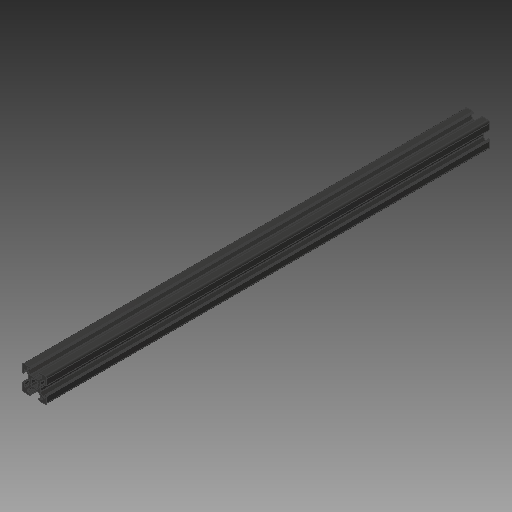
# Autodesk Inventor part: Profile horizontal 20x20x360
Saved by Autodesk Inventor 2017 (Build 210142000, 142)
## iProperties
Company: FABLAB Frenchmakers
Part Number: Profile horizontal 20x20x360
Material: Aluminium
Document SubType Name: Modeling
Designer: FABLAB Frenchmakers
Density: 2.7 g/cm^3
Appearance: Aluminium - Plat(1)
Mass: 157.502 g
Surface Area: 633.6 cm^2
Volume: 58.3342 cm^3
Stock Number: 1420-01-03
Project: 1420 Vauban 3D XL
Catalog Web Link: http://frenchmakers.com/
Autodesk Inventor part; units mm, degrees
ref_plane "YZ Plane" through (0, 0, 0) normal (1, 0, 0) x (0, 1, 0)
ref_plane "XZ Plane" through (0, 0, 0) normal (0, 1, 0) x (-1, 0, 0)
ref_plane "XY Plane" through (0, 0, 0) normal (0, 0, 1) x (1, 0, 0)
sketch "Esquisse1" plane through (0, 0, 0) normal (0, 0, 1) x (1, 0, 0)
  arc A0 (10, 8.5) -> (8.5, 10) centre (8.5, 8.5) ccw
  line L0 (3.85, 10) -> (8.5, 10)
  arc A1 (3.85, 10) -> (3.65, 9.8) centre (3.85, 9.8) ccw
  line L1 (3.65, 9.5) -> (3.65, 9.8)
  line L2 (3.3, 9.5) -> (3.65, 9.5)
  arc A2 (3.3, 9.5) -> (3.1, 9.3) centre (3.3, 9.3) ccw
  line L3 (3.1, 9) -> (3.1, 9.3)
  arc A3 (3.1, 9) -> (3.6, 8.5) centre (3.6, 9) ccw
  line L4 (5.5, 8.5) -> (3.6, 8.5)
  arc A4 (6, 8) -> (5.5, 8.5) centre (5.5, 8) ccw
  line L5 (6, 7.2678) -> (6, 8)
  arc A5 (5.8536, 6.9142) -> (6, 7.2678) centre (5.5, 7.2678) ccw
  line L6 (3.5858, 4.6464) -> (5.8536, 6.9142)
  arc A6 (3.2322, 4.5) -> (3.5858, 4.6464) centre (3.2322, 5) ccw
  line L7 (0.9536, 4.5) -> (3.2322, 4.5)
  arc A7 (0.9536, 4.5) -> (0.8536, 4.4732) centre (0.9536, 4.3) ccw
  line L8 (0.1, 4.0381) -> (0.8536, 4.4732)
  arc A8 (-0.1, 4.0381) -> (0.1, 4.0381) centre (0, 4.2113) ccw
  line L9 (-0.8536, 4.4732) -> (-0.1, 4.0381)
  arc A9 (-0.8536, 4.4732) -> (-0.9536, 4.5) centre (-0.9536, 4.3) ccw
  line L10 (-3.2322, 4.5) -> (-0.9536, 4.5)
  arc A10 (-3.5858, 4.6464) -> (-3.2322, 4.5) centre (-3.2322, 5) ccw
  line L11 (-5.8536, 6.9142) -> (-3.5858, 4.6464)
  arc A11 (-6, 7.2678) -> (-5.8536, 6.9142) centre (-5.5, 7.2678) ccw
  line L12 (-6, 8) -> (-6, 7.2678)
  arc A12 (-5.5, 8.5) -> (-6, 8) centre (-5.5, 8) ccw
  line L13 (-3.6, 8.5) -> (-5.5, 8.5)
  arc A13 (-3.6, 8.5) -> (-3.1, 9) centre (-3.6, 9) ccw
  line L14 (-3.1, 9.3) -> (-3.1, 9)
  arc A14 (-3.1, 9.3) -> (-3.3, 9.5) centre (-3.3, 9.3) ccw
  line L15 (-3.65, 9.5) -> (-3.3, 9.5)
  line L16 (-3.65, 9.8) -> (-3.65, 9.5)
  arc A15 (-3.65, 9.8) -> (-3.85, 10) centre (-3.85, 9.8) ccw
  line L17 (-8.5, 10) -> (-3.85, 10)
  arc A16 (-8.5, 10) -> (-10, 8.5) centre (-8.5, 8.5) ccw
  line L18 (-10, 3.85) -> (-10, 8.5)
  arc A17 (-10, 3.85) -> (-9.8, 3.65) centre (-9.8, 3.85) ccw
  line L19 (-9.5, 3.65) -> (-9.8, 3.65)
  line L20 (-9.5, 3.3) -> (-9.5, 3.65)
  arc A18 (-9.5, 3.3) -> (-9.3, 3.1) centre (-9.3, 3.3) ccw
  line L21 (-9, 3.1) -> (-9.3, 3.1)
  arc A19 (-9, 3.1) -> (-8.5, 3.6) centre (-9, 3.6) ccw
  line L22 (-8.5, 5.5) -> (-8.5, 3.6)
  arc A20 (-8, 6) -> (-8.5, 5.5) centre (-8, 5.5) ccw
  line L23 (-7.2678, 6) -> (-8, 6)
  arc A21 (-6.9142, 5.8536) -> (-7.2678, 6) centre (-7.2678, 5.5) ccw
  line L24 (-4.6464, 3.5858) -> (-6.9142, 5.8536)
  arc A22 (-4.5, 3.2322) -> (-4.6464, 3.5858) centre (-5, 3.2322) ccw
  line L25 (-4.5, 0.9536) -> (-4.5, 3.2322)
  arc A23 (-4.5, 0.9536) -> (-4.4732, 0.8536) centre (-4.3, 0.9536) ccw
  line L26 (-4.0381, 0.1) -> (-4.4732, 0.8536)
  arc A24 (-4.0381, -0.1) -> (-4.0381, 0.1) centre (-4.2113, 0) ccw
  line L27 (-4.4732, -0.8536) -> (-4.0381, -0.1)
  arc A25 (-4.4732, -0.8536) -> (-4.5, -0.9536) centre (-4.3, -0.9536) ccw
  line L28 (-4.5, -3.2322) -> (-4.5, -0.9536)
  arc A26 (-4.6464, -3.5858) -> (-4.5, -3.2322) centre (-5, -3.2322) ccw
  line L29 (-6.9142, -5.8536) -> (-4.6464, -3.5858)
  arc A27 (-7.2678, -6) -> (-6.9142, -5.8536) centre (-7.2678, -5.5) ccw
  line L30 (-8, -6) -> (-7.2678, -6)
  arc A28 (-8.5, -5.5) -> (-8, -6) centre (-8, -5.5) ccw
  line L31 (-8.5, -3.6) -> (-8.5, -5.5)
  arc A29 (-8.5, -3.6) -> (-9, -3.1) centre (-9, -3.6) ccw
  line L32 (-9.3, -3.1) -> (-9, -3.1)
  arc A30 (-9.3, -3.1) -> (-9.5, -3.3) centre (-9.3, -3.3) ccw
  line L33 (-9.5, -3.65) -> (-9.5, -3.3)
  line L34 (-9.8, -3.65) -> (-9.5, -3.65)
  arc A31 (-9.8, -3.65) -> (-10, -3.85) centre (-9.8, -3.85) ccw
  line L35 (-10, -8.5) -> (-10, -3.85)
  arc A32 (-10, -8.5) -> (-8.5, -10) centre (-8.5, -8.5) ccw
  line L36 (-3.85, -10) -> (-8.5, -10)
  arc A33 (-3.85, -10) -> (-3.65, -9.8) centre (-3.85, -9.8) ccw
  line L37 (-3.65, -9.5) -> (-3.65, -9.8)
  line L38 (-3.3, -9.5) -> (-3.65, -9.5)
  arc A34 (-3.3, -9.5) -> (-3.1, -9.3) centre (-3.3, -9.3) ccw
  line L39 (-3.1, -9) -> (-3.1, -9.3)
  arc A35 (-3.1, -9) -> (-3.6, -8.5) centre (-3.6, -9) ccw
  line L40 (-5.5, -8.5) -> (-3.6, -8.5)
  arc A36 (-6, -8) -> (-5.5, -8.5) centre (-5.5, -8) ccw
  line L41 (-6, -7.2678) -> (-6, -8)
  arc A37 (-5.8536, -6.9142) -> (-6, -7.2678) centre (-5.5, -7.2678) ccw
  line L42 (-3.5858, -4.6464) -> (-5.8536, -6.9142)
  arc A38 (-3.2322, -4.5) -> (-3.5858, -4.6464) centre (-3.2322, -5) ccw
  line L43 (-0.9536, -4.5) -> (-3.2322, -4.5)
  arc A39 (-0.9536, -4.5) -> (-0.8536, -4.4732) centre (-0.9536, -4.3) ccw
  line L44 (-0.1, -4.0381) -> (-0.8536, -4.4732)
  arc A40 (0.1, -4.0381) -> (-0.1, -4.0381) centre (0, -4.2113) ccw
  line L45 (0.8536, -4.4732) -> (0.1, -4.0381)
  arc A41 (0.8536, -4.4732) -> (0.9536, -4.5) centre (0.9536, -4.3) ccw
  line L46 (3.2322, -4.5) -> (0.9536, -4.5)
  arc A42 (3.5858, -4.6464) -> (3.2322, -4.5) centre (3.2322, -5) ccw
  line L47 (5.8536, -6.9142) -> (3.5858, -4.6464)
  arc A43 (6, -7.2678) -> (5.8536, -6.9142) centre (5.5, -7.2678) ccw
  line L48 (6, -8) -> (6, -7.2678)
  arc A44 (5.5, -8.5) -> (6, -8) centre (5.5, -8) ccw
  line L49 (3.6, -8.5) -> (5.5, -8.5)
  arc A45 (3.6, -8.5) -> (3.1, -9) centre (3.6, -9) ccw
  line L50 (3.1, -9.3) -> (3.1, -9)
  arc A46 (3.1, -9.3) -> (3.3, -9.5) centre (3.3, -9.3) ccw
  line L51 (3.65, -9.5) -> (3.3, -9.5)
  line L52 (3.65, -9.8) -> (3.65, -9.5)
  arc A47 (3.65, -9.8) -> (3.85, -10) centre (3.85, -9.8) ccw
  line L53 (8.5, -10) -> (3.85, -10)
  arc A48 (8.5, -10) -> (10, -8.5) centre (8.5, -8.5) ccw
  line L54 (10, -3.85) -> (10, -8.5)
  arc A49 (10, -3.85) -> (9.8, -3.65) centre (9.8, -3.85) ccw
  line L55 (9.5, -3.65) -> (9.8, -3.65)
  line L56 (9.5, -3.3) -> (9.5, -3.65)
  arc A50 (9.5, -3.3) -> (9.3, -3.1) centre (9.3, -3.3) ccw
  line L57 (9, -3.1) -> (9.3, -3.1)
  arc A51 (9, -3.1) -> (8.5, -3.6) centre (9, -3.6) ccw
  line L58 (8.5, -5.5) -> (8.5, -3.6)
  arc A52 (8, -6) -> (8.5, -5.5) centre (8, -5.5) ccw
  line L59 (7.2678, -6) -> (8, -6)
  arc A53 (6.9142, -5.8536) -> (7.2678, -6) centre (7.2678, -5.5) ccw
  line L60 (4.6464, -3.5858) -> (6.9142, -5.8536)
  arc A54 (4.5, -3.2322) -> (4.6464, -3.5858) centre (5, -3.2322) ccw
  line L61 (4.5, -0.9536) -> (4.5, -3.2322)
  arc A55 (4.5, -0.9536) -> (4.4732, -0.8536) centre (4.3, -0.9536) ccw
  line L62 (4.0381, -0.1) -> (4.4732, -0.8536)
  arc A56 (4.0381, 0.1) -> (4.0381, -0.1) centre (4.2113, 0) ccw
  line L63 (4.4732, 0.8536) -> (4.0381, 0.1)
  arc A57 (4.4732, 0.8536) -> (4.5, 0.9536) centre (4.3, 0.9536) ccw
  line L64 (4.5, 3.2322) -> (4.5, 0.9536)
  arc A58 (4.6464, 3.5858) -> (4.5, 3.2322) centre (5, 3.2322) ccw
  line L65 (6.9142, 5.8536) -> (4.6464, 3.5858)
  arc A59 (7.2678, 6) -> (6.9142, 5.8536) centre (7.2678, 5.5) ccw
  line L66 (8, 6) -> (7.2678, 6)
  arc A60 (8.5, 5.5) -> (8, 6) centre (8, 5.5) ccw
  line L67 (8.5, 3.6) -> (8.5, 5.5)
  arc A61 (8.5, 3.6) -> (9, 3.1) centre (9, 3.6) ccw
  line L68 (9.3, 3.1) -> (9, 3.1)
  arc A62 (9.3, 3.1) -> (9.5, 3.3) centre (9.3, 3.3) ccw
  line L69 (9.5, 3.65) -> (9.5, 3.3)
  line L70 (9.8, 3.65) -> (9.5, 3.65)
  arc A63 (9.8, 3.65) -> (10, 3.85) centre (9.8, 3.85) ccw
  line L71 (10, 8.5) -> (10, 3.85)
  arc A64 (2.9922, 1.9099) -> (1.9139, 2.9896) centre (0, 0) ccw
  line L72 (2.9922, 1.9099) -> (2.4453, 1.2582)
  arc A65 (2.4453, -1.2582) -> (2.4453, 1.2582) centre (0, 0) ccw
  line L73 (2.4453, -1.2582) -> (2.9922, -1.9099)
  arc A66 (1.9139, -2.9896) -> (2.9922, -1.9099) centre (0, 0) ccw
  line L74 (1.9139, -2.9896) -> (1.2582, -2.4453)
  arc A67 (-1.2582, -2.4453) -> (1.2582, -2.4453) centre (0, 0) ccw
  line L75 (-1.2582, -2.4453) -> (-1.9139, -2.9896)
  arc A68 (-2.9922, -1.9099) -> (-1.9139, -2.9896) centre (0, 0) ccw
  line L76 (-2.9922, -1.9099) -> (-2.4453, -1.2582)
  arc A69 (-2.4453, 1.2582) -> (-2.4453, -1.2582) centre (0, 0) ccw
  line L77 (-2.4453, 1.2582) -> (-2.9922, 1.9099)
  arc A70 (-1.9139, 2.9896) -> (-2.9922, 1.9099) centre (0, 0) ccw
  line L78 (-1.9139, 2.9896) -> (-1.2582, 2.4453)
  arc A71 (1.2582, 2.4453) -> (-1.2582, 2.4453) centre (0, 0) ccw
  line L79 (1.2582, 2.4453) -> (1.9139, 2.9896)
  point P0 (8.5, -10)
  constraints: 160 end point, 144 point on circle, 72 centre point
extrude "Extrusion1" add sketch "Esquisse1" along normal mid plane 360
